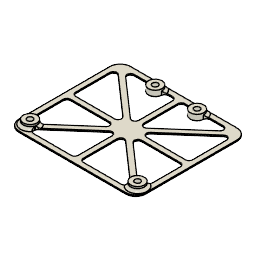
LCC Lighting Controller Mount v1 (Autodesk Fusion 360 design; units mm, degrees)
Autodesk Fusion 360 part; units mm, degrees
sketch "Sketch1" plane through (0, 0, 0) normal (0, 1, 0) x (1, 0, 0)
  line L0 (31, -32.5) -> (-31, -32.5)
  line L1 (-37, -26.5) -> (-37, 26.5)
  line L2 (-31, 32.5) -> (31, 32.5)
  line L3 (37, 26.5) -> (37, -26.5)
  line L4 (37, -32.5) -> (-37, 32.5) construction
  line L5 (-37, -32.5) -> (37, 32.5) construction
  arc A0 (-31, 32.5) -> (-37, 26.5) centre (-31, 26.5) ccw
  arc A1 (37, 26.5) -> (31, 32.5) centre (31, 26.5) ccw
  arc A2 (31, -32.5) -> (37, -26.5) centre (31, -26.5) ccw
  arc A3 (-37, -26.5) -> (-31, -32.5) centre (-31, -26.5) ccw
  circle A4 centre (-31.25, -25.7) radius 1.625
  circle A5 centre (31.25, -25.7) radius 4
  circle A6 centre (-31.25, -25.7) radius 4
  circle A7 centre (31.25, -25.7) radius 1.625
  circle A8 centre (-12.15, 28) radius 4
  circle A9 centre (-12.15, 28) radius 1.625
  circle A10 centre (12.15, 28) radius 1.625
  circle A11 centre (12.15, 28) radius 4
  arc A12 (31, -29.5) -> (34, -26.5) centre (31, -26.5) ccw
  line L6 (34, 26.5) -> (34, -26.5)
  arc A13 (34, 26.5) -> (31, 29.5) centre (31, 26.5) ccw
  line L7 (-31, 29.5) -> (31, 29.5)
  arc A14 (-31, 29.5) -> (-34, 26.5) centre (-31, 26.5) ccw
  line L8 (-34, -26.5) -> (-34, 26.5)
  arc A15 (-34, -26.5) -> (-31, -29.5) centre (-31, -26.5) ccw
  line L9 (31, -29.5) -> (-31, -29.5)
  line L10 (54.1979, -45.6097) -> (-51.5836, 47.3064)
  line L11 (-51.3223, -47.0769) -> (53.9362, 45.3799)
  line L12 (-53.9385, -45.382) -> (51.3202, 47.075)
  line L13 (51.5836, -47.3064) -> (-54.1979, 45.6097)
  line L14 (0, -29.5) -> (0, 29.5) construction
  line L15 (34, 0) -> (-34, 0) construction
  line L16 (37, 1.5) -> (-45.8026, 1.5)
  line L17 (37, -1.5) -> (-45.7365, -1.5)
  line L18 (1.5, -55.0004) -> (1.5, 54.9997)
  line L19 (-1.5, -55.0004) -> (-1.5, 54.9997)
  dimension "d1" = 74
  dimension "d2" = 65
  dimension "d3" = 6
  dimension "d4" = 3.25
  dimension "d5" = 8
  dimension "d6" = 62.5
  dimension "d7" = 31.25
  dimension "d8" = 6.8
  dimension "d9" = 4.5
  dimension "d10" = 24.3
  dimension "d11" = 12.15
  dimension "d12" = 3
  dimension "d13" = 1.5
  dimension "d14" = 1.5
  dimension "d15" = -1.5
  dimension "d16" = -1.5
  dimension "d17" = 1.5
  dimension "d18" = -1.5
  dimension "d19" = 1.5
  dimension "d20" = -1.5
  constraint horizontal L0
  constraint perpendicular L0 L1
  constraint parallel L0 L2
  constraint parallel L1 L3
  constraint coincident L4 origin
  constraint coincident L5 origin
  constraint coincident L4.end L1
  constraint coincident L4.end L2
  constraint tangent L1 A0
  constraint tangent L2 A0
  constraint coincident L5.end L2
  constraint coincident L5.end L3
  constraint tangent L2 A1
  constraint tangent L3 A1
  constraint equal A0 A1
  constraint coincident L4.start L3
  constraint coincident L4.start L0
  constraint tangent L3 A2
  constraint tangent L0 A2
  constraint equal A0 A2
  constraint coincident L5.start L1
  constraint coincident L5.start L0
  constraint tangent L1 A3
  constraint tangent L0 A3
  constraint equal A0 A3
  constraint concentric A4 A6
  constraint concentric A5 A7
  constraint equal A5 A6
  constraint equal A4 A7
  constraint horizontal A4.centre A5.centre
  constraint concentric A8 A9
  constraint concentric A10 A11
  constraint equal A8 A11
  constraint equal A5 A11
  constraint equal A7 A10
  constraint equal A9 A10
  constraint horizontal A8.centre A10.centre
  constraint midpoint L9 L14.start
  constraint midpoint L7 L14.end
  constraint midpoint L6 L15.start
  constraint midpoint L8 L15.end
  constraint coincident L3 L16.start
  constraint coincident L3 L17.start
  measures "d1" distance of L4.end L5.end
  measures "d2" distance of L5.start L4.end
  measures "d3" radius of A0
  measures "d4" diameter of A4
  measures "d5" diameter of A6
  measures "d6" distance of A5.centre A4.centre
  measures "d7" horizontal distance of origin A4.centre
  measures "d8" distance of L0 A5.centre
  measures "d9" distance of L2 A10.centre
  measures "d10" distance of A8.centre A10.centre
  measures "d11" horizontal distance of origin A8.centre
extrude "Extrude1" add sketch "Sketch1" along normal blind 1 contours L0 A2 A5 L9 L13 L18 | L0 L9 L18 L19 | A2 A5 L10 L13 | L0 A3 A6 L9 L11 L19 | L9 L11 L13 L18 L19 | L3 A2 A5 L6 L10 L17 | A5 A12 L10 L13 | A5 A12 L9 L13 | A5 A12 L9 L13 | A5 L10 L13 L17 L18 | L11 L13 L17 L18 | A5 A12 L6 L10 | A5 A7 A12 L10 L13 | A3 A6 L11 L12 | A6 A15 L9 L11 | A6 A15 L9 L11 | L11 L13 L17 L19 | A6 L11 L12 L17 L19 | L11 L13 L17 | L10 L11 L17 L18 | L11 L17 L18 | L3 L6 L16 L17 | A5 A7 A12 L6 L10 | L1 A3 A6 L8 L12 L17 | A6 A15 L11 L12 | A4 A6 A15 L11 L12 | L13 L17 L19 | L12 L13 L17 L19 | L10 L11 L12 L13 L16 L17 L18 L19 | L6 L10 L11 L16 L17 | L10 L11 L18 | L3 A1 L6 A13 L11 L16 | A6 L8 A15 L12 | L8 L12 L13 L16 L17 | L12 L13 L19 | L10 L11 L16 L18 | L10 L16 L18 | L1 L8 L16 L17 | A4 A6 L8 A15 L12 | L12 L13 L16 L19 | L12 L16 L19 | A13 L11 L12 L16 L18 | L10 L12 L16 | L10 L12 L16 L18 | A1 A13 L11 L12 | L1 A0 A14 L8 L13 L16 | A14 L10 L13 L16 L19 | L10 L12 L16 L19 | L7 L10 L12 L18 L19 | L2 A1 A11 A13 L7 L12 L18 | A0 A14 L10 L13 | L2 L7 L18 L19 | L2 A0 A8 L7 A14 L10 L19 | A10 A11 L7 | A10 A11 L7 | A8 A9 L7 | A8 A9 L7
extrude "Extrude2" add sketch "Sketch1" along normal blind 3.5 contours A5 A12 L10 L13 | A5 A12 L9 L13 | A5 A12 L9 L13 | A5 A12 L6 L10 | A5 A7 A12 L10 L13 | A6 A15 L9 L11 | A6 A15 L9 L11 | A5 A7 A12 L6 L10 | A6 A15 L11 L12 | A4 A6 A15 L11 L12 | A6 L8 A15 L12 | A4 A6 L8 A15 L12 | A10 A11 L7 | A10 A11 L7 | A8 A9 L7 | A8 A9 L7
fillet "Fillet1" radius 2 32 edges at (-8.4419, 0.5, -29.5) (-15.8581, 0.5, -29.5) (-1.5, 0.5, -29.5) (1.5, 0.5, -29.5) (-31.2951, 0.5, -29.4854) (8.4419, 0.5, -29.5) (15.8581, 0.5, -29.5) (31.2951, 0.5, -29.4854) (-1.5, 0.5, -3.3141) (1.5, 0.5, -3.3141) (3.9806, 0.5, -1.5) (-3.9806, 0.5, -1.5) (-3.9806, 0.5, 1.5) (-1.5, 0.5, 3.3141) (1.5, 0.5, 3.3141) (3.9806, 0.5, 1.5) (34, 0.5, 1.5) (34, 0.5, -1.5) (-34, 0.5, -1.5) (-34, 0.5, 1.5) (-30.001, 0.5, 29.5) (-34, 0.5, 22.7953) (-28.3705, 0.5, 22.9236) (-27.2571, 0.5, 25.9386) (-1.5, 0.5, 29.5) (1.5, 0.5, 29.5) (34, 0.5, 22.7953) (28.3705, 0.5, 22.9236) (27.2571, 0.5, 25.9386) (30.001, 0.5, 29.5) (-33.7656, 0.5, -27.6625) (33.7656, 0.5, -27.6625)
fillet "Fillet2" radius 1.5 6 edges at (-27.6336, 1, 23.9907) (-34.3204, 1, 28.2637) (27.6336, 1, 23.9907) (34.3204, 1, 28.2637) (-12.15, 1, -32) (12.15, 1, -32)
chamfer "Chamfer1" distance 0.3 angle 45 1 faces at (0.8918, 0, 1.9703)
equation "d7 = d6 / 2"
equation "d11 = d10 / 2"
